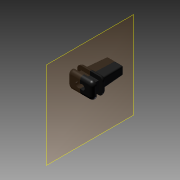
# Autodesk Inventor part: 276-2177-018 Rev1
Saved by Autodesk Inventor 2016 SP2 (Build 200236200, 236)
## iProperties
Category: Motors
Company: Autodesk Inc.
Created: 2012-01-23
Part Number: 276-2177-018 Rev1
Material: Rubber
Document SubType Name: Modeling
Designer: Autodesk Inc.
Density: 0.93 g/cm^3
Catalog Web Link: http://www.vexrobotics.com/276-2181.html
Vendor: VEX
Mass: 0.084435 g
Surface Area: 2.41868 cm^2
Volume: 0.0907903 cm^3
Appearance: Glossy - Black
Author: Autodesk Inc.
Autodesk Inventor part; units mm, degrees
sketch "Sketch1" plane through (0, 0, 0) normal (0, 0, 1) x (1, 0, 0)
  line L0 (2.2, -2.1) -> (-2.2, -2.1)
  spline S0 degree 3 poles (3.2, -1.1) (3.2, -1.5502) (2.8577, -1.9776) (2.4183, -2.0759) (2.3467, -2.0919) (2.2734, -2.1) (2.2, -2.1) knots 0 0 0 0 0.859892 0.859892 0.859892 1 1 1 1
  line L1 (3.2, 1.1) -> (3.2, -1.1)
  spline S1 degree 3 poles (2.2, 2.1) (2.6502, 2.1) (3.0776, 1.7577) (3.1759, 1.3183) (3.1919, 1.2467) (3.2, 1.1734) (3.2, 1.1) knots 0 0 0 0 0.859892 0.859892 0.859892 1 1 1 1
  line L2 (-2.2, 2.1) -> (2.2, 2.1)
  arc A0 (-2.2, 2.1) -> (-3.2, 1.1) centre (-2.2, 1.1) ccw
  line L3 (-3.2, -1.1) -> (-3.2, 1.1)
  arc A1 (-3.2, -1.1) -> (-2.2, -2.1) centre (-2.2, -1.1) ccw
  line L4 (-2.2, -1.1) -> (2.2, -1.1)
  line L5 (-2.2, 1.1) -> (-2.2, -1.1)
  line L6 (2.2, 1.1) -> (-2.2, 1.1)
  line L7 (2.2, -1.1) -> (2.2, 1.1)
  point P0 (0, 0)
  point P1 (0, 0)
  constraints: 16 end point, 4 point on circle, 2 centre point, 6 other
extrude "Extrusion1" add sketch "Sketch1" along normal blind 0.9906 contours L0 A1 L3 A0 L2 S1 L1 S0 | L5 L6 L7 L4
extrude "Extrusion2" add sketch "Sketch1" against normal blind 1.4986 contours L5 L6 L7 L4
fillet "Fillet1" radius 0.8636 8 edges at (2.902, 1.801, 0.9906) (3.2, 0, 0.9906) (2.901, -1.802, 0.9906) (0, -2.1, 0.9906) (-2.9071, -1.8071, 0.9906) (-3.2, 0, 0.9906) (-2.9071, 1.8071, 0.9906) (0, 2.1, 0.9906)
ref_plane "Work Plane1" through (0, 0, -0.7493) normal (0, 0, -1) x (-1, 0, 0)
mirror "Mirror1" about plane through (0, 0, -0.7493) normal (0, 0, -1) of "Extrusion1", "Fillet1"
sketch "Sketch2" plane through (2.2, -1.2364, -2.4892) normal (0, 0, -1) x (-1, 0, 0)
  line L0 (-0.1364, 2.3364) -> (-0.1364, 0.1364) projected
  line L1 (0, 0) -> (4.4, 0) projected
  line L2 (4.5364, 0.1364) -> (4.5364, 2.3364) projected
  line L3 (4.4, 2.4728) -> (0, 2.4728) projected
  line L4 (0.1811, 2.4728) -> (4.2189, 2.4728)
  line L5 (4.5364, 2.1553) -> (4.5364, 0.3175)
  line L6 (4.2189, 0) -> (0.1811, 0)
  line L7 (-0.1364, 0.3175) -> (-0.1364, 2.1553)
  arc A0 (0.1811, 2.4728) -> (-0.1364, 2.1553) centre (0.1811, 2.1553) ccw
  arc A1 (4.5364, 2.1553) -> (4.2189, 2.4728) centre (4.2189, 2.1553) ccw
  arc A2 (4.2189, 0) -> (4.5364, 0.3175) centre (4.2189, 0.3175) ccw
  arc A3 (-0.1364, 0.3175) -> (0.1811, 0) centre (0.1811, 0.3175) ccw
  point P0 (2.2, 1.2364)
  point P1 (-0.1364, 2.4728)
  point P2 (4.5364, 0)
  point P3 (4.5364, 2.4728)
  point P4 (-0.1364, 0)
  dimension "d16" = 0.3175
  constraints: 8 end point, 8 point on circle, 8 point on line, 8 tangent, 4 centre point, 4 collinear, 3 equal radius, 2 parallel, 1 horizontal, 1 perpendicular
  measures "d16" radius of A0
ref_plane "Work Plane3" through (2.2, -1.2364, -7.8994) normal (0, 0, -1) x (-1, 0, 0)
sketch "Sketch3" plane through (2.2, -1.2364, -7.8994) normal (0, 0, -1) x (-1, 0, 0)
  point P0 (2.2, 1.2364)
ref_plane "Work Plane4" through (2.2, -1.2364, -7.8994) normal (0, 0, -1) x (-1, 0, 0)
sketch "Sketch4" plane through (2.2, -1.2364, -7.8994) normal (0, 0, -1) x (-1, 0, 0)
  line L0 (0.4855, 0.2077) -> (3.9145, 0.2077)
  line L1 (4.232, 0.5252) -> (4.232, 1.9476)
  line L2 (3.9145, 2.2651) -> (0.4855, 2.2651)
  line L3 (0.168, 1.9476) -> (0.168, 0.5252)
  line L4 (4.4, 2.4728) -> (0, 2.4728) projected
  line L5 (-0.1364, 2.3364) -> (-0.1364, 0.1364) projected
  arc A0 (0.4855, 2.2651) -> (0.168, 1.9476) centre (0.4855, 1.9476) ccw
  arc A1 (4.232, 1.9476) -> (3.9145, 2.2651) centre (3.9145, 1.9476) ccw
  arc A2 (3.9145, 0.2077) -> (4.232, 0.5252) centre (3.9145, 0.5252) ccw
  arc A3 (0.168, 0.5252) -> (0.4855, 0.2077) centre (0.4855, 0.5252) ccw
  point P0 (2.2, 1.2364)
  point P1 (0.168, 0.2077)
  point P2 (4.232, 2.2651)
  point P3 (4.232, 0.2077)
  point P4 (0.168, 2.2651)
  point P5 (2.2, 2.2651)
  point P6 (2.2, 2.4728)
  point P7 (0.168, 1.2364)
  point P8 (-0.1364, 1.2364)
  dimension "d7" = 4.064
  dimension "d8" = 2.0574
  dimension "d17" = 0.3175
  constraints: 8 end point, 8 point on circle, 8 point on line, 8 tangent, 4 centre point, 4 midpoint, 3 equal radius, 2 parallel, 1 horizontal, 1 horizontal alignment, 1 perpendicular, 1 vertical alignment
  measures "d7" distance of point (4.232, 2.265) point (0.168, 2.265)
  measures "d8" distance of point (4.232, 0.208) point (4.232, 2.265)
  measures "d17" radius of A0
loft "Loft1" add profiles "Sketch2", "Sketch4"
sketch "Sketch5" plane through (0, 0, 0.9906) normal (0, 0, 1) x (1, 0, 0)
  arc A0 (-0.2174, 0.5853) -> (-0.2174, -0.5853) centre (-0.5, 0) ccw
  arc A1 (-0.2174, 0.5853) -> (0.2174, 0.5853) centre (0, 1.0356) ccw
  arc A2 (0.2174, -0.5853) -> (0.2174, 0.5853) centre (0.5, 0) ccw
  arc A3 (0.2174, -0.5853) -> (-0.2174, -0.5853) centre (0, -1.0356) ccw
  point P0 (0, 0)
  point P1 (0, 0)
  constraints: 8 point on circle, 4 centre point
extrude "Extrusion3" cut sketch "Sketch5" against normal up to next
fillet "Fillet3" radius 0.3124 8 edges at (-1.939, 0.9357, -7.8994) (-2.032, 0, -7.8994) (-1.939, -0.9357, -7.8994) (0, -1.0287, -7.8994) (1.939, -0.9357, -7.8994) (2.032, 0, -7.8994) (1.939, 0.9357, -7.8994) (0, 1.0287, -7.8994)
ref_plane "Work Plane5" through (0, -2.1, -1.4986) normal (-1, 0, 0) x (0, -1, 0)
body "Solid1"
